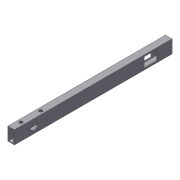
# Autodesk Inventor part: FrameSideRail
Saved by Autodesk Inventor 2012 (Build 160160000, 160)
## iProperties
Created: 2013-01-06
Part Number: FrameSideRail
Material: Aluminum-6061
Document SubType Name: Modeling
Designer: JesseK
Density: 2.71 g/cm^3
Mass: 661.381 g
Surface Area: 1597.58 cm^2
Volume: 244.052 cm^3
Author: JesseK
Autodesk Inventor part; units mm, degrees
ref_plane "YZ Plane" through (0, 0, 0) normal (1, 0, 0) x (0, 1, 0)
ref_plane "XZ Plane" through (0, 0, 0) normal (0, 1, 0) x (-1, 0, 0)
ref_plane "XY Plane" through (0, 0, 0) normal (0, 0, 1) x (1, 0, 0)
sketch "Sketch1" plane through (0, 0, 0) normal (0, 0, 1) x (1, 0, 0)
  line L0 (0, 0) -> (25.4, 0)
  line L1 (25.4, 0) -> (25.4, 50.8)
  line L2 (25.4, 50.8) -> (0, 50.8)
  line L3 (0, 50.8) -> (0, 0)
  line L4 (3.175, 3.175) -> (22.225, 3.175)
  line L5 (22.225, 3.175) -> (22.225, 47.625)
  line L6 (22.225, 47.625) -> (3.175, 47.625)
  line L7 (3.175, 47.625) -> (3.175, 3.175)
  dimension "d0" = 25.4
  dimension "d1" = 50.8
  dimension "d2" = 19.05
  dimension "d3" = 44.45
  dimension "d4" = 3.175
  dimension "d5" = 3.175
  constraints: 16 end point, 4 parallel, 2 horizontal, 2 perpendicular
  measures "d0" distance of L0.start L0.end
  measures "d1" distance of L2.end L0.start
  measures "d2" distance between parallel lines of L5 L7
  measures "d3" distance between parallel lines of L4 L6
  measures "d4" distance between parallel lines of L3 L7
  measures "d5" distance between parallel lines of L0 L4
extrude "Extrusion1" add sketch "Sketch1" along normal blind 609.6
sketch "Sketch2" plane through (25.4, 0, 0) normal (1, 0, 0) x (0, 0, -1)
  line L0 (-609.6, 50.8) -> (-609.6, 0) projected
  line L1 (0, 0) -> (0, 50.8) projected
  line L2 (-57.15, 44.45) -> (-107.95, 44.45)
  line L3 (-107.95, 44.45) -> (-107.95, 6.35)
  line L4 (-107.95, 6.35) -> (-57.15, 6.35)
  line L5 (-57.15, 6.35) -> (-57.15, 44.45)
  line L6 (0, 0) -> (-609.6, 0) projected
  line L7 (0, 25.4) -> (0, 0)
  circle A0 centre (-533.4, 25.4) radius 14.2875
  dimension "d12" = 57.15
  dimension "d21" = 107.95
  dimension "d29" = 50.8
  dimension "d32" = 38.1
  dimension "d33" = 6.35
  dimension "d64" = 28.575
  dimension "d65" = 76.2
  dimension "d66" = 25.4
  constraints: 10 end point, 2 parallel, 1 centre point, 1 horizontal, 1 midpoint, 1 perpendicular, 1 vertical
  measures "d12" distance between parallel lines of L1 L5
  measures "d21" distance between parallel lines of L3 L1
  measures "d29" distance of L2.start L2.end
  measures "d32" distance of L2.end L3.end
  measures "d33" distance between parallel lines of L6 L4
  measures "d64" diameter of A0
  measures "d65" distance from line of A0.centre L0
  measures "d66" distance from line of L6 A0.centre
extrude "Extrusion2" cut sketch "Sketch2" against normal through all
sketch "Sketch5" plane through (0, 0, 0) normal (0, -1, 0) x (1, 0, 0)
  line L0 (25.4, 609.6) -> (0, 609.6) projected
  line L1 (25.4, 0) -> (25.4, 609.6) projected
  circle A0 centre (12.7, 571.5) radius 3.175
  circle A1 centre (12.7, 495.3) radius 3.175
  dimension "d53" = 38.1
  dimension "d54" = 76.2
  dimension "d55" = 12.7
  dimension "d56" = 12.7
  dimension "d57" = 6.35
  constraints: 2 centre point, 1 equal radius
  measures "d53" distance from line of L0 A0.centre
  measures "d54" distance of A1.centre A0.centre
  measures "d55" distance from line of L1 A0.centre
  measures "d56" distance from line of L1 A1.centre
  measures "d57" diameter of A1
extrude "Extrusion5" cut sketch "Sketch5" against normal through all
sketch "Sketch6" plane through (0, 50.8, 0) normal (0, 1, 0) x (1, 0, 0)
  circle A0 centre (12.7, -495.3) radius 3.175 projected
  circle A1 centre (12.7, -571.5) radius 3.175 projected
  circle A2 centre (12.7, -495.3) radius 6.35
  circle A3 centre (12.7, -571.5) radius 6.35
  dimension "d60" = 12.7
  dimension "d61" = 12.7
  constraints: 2 centre point, 2 coincident
  measures "d60" diameter of A3
  measures "d61" diameter of A2
extrude "Extrusion6" cut sketch "Sketch6" against normal up to next
body "Solid1"
